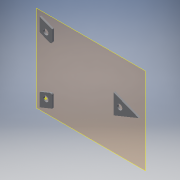
# Autodesk Inventor part: Orelhinhas
Saved by Autodesk Inventor 2019 (Build 230136000, 136)
## iProperties
Created: 2020-05-31
Part Number: Orelhinhas
Material: Genérico
Document SubType Name: Modeling
Designer: lukas
Density: 1 g/cm^3
Appearance: Padrão
Categories: <MemberInstance><Categories><Category DisplayName="" Mnemonic="CABLEANDHARNESS" InternalName="e4a7e005-5e42-4d16-b293-125e7f0d0512"><Category DisplayName="" Mnemonic="CONNECTORS" InternalName="6f634eba-a678-4820-a31d-2c2d5ee6728e"><CategoryParameter DisplayName="" Mnemonic="REFDES" InternalName="c3740e8c-60ab-4d5d-8584-52b73222f2f0"/><Category DisplayName="" Mnemonic="DISCRETEWIRE" InternalName="9a3407de-09b2-4cdb-8c40-9708d5144a28"/></Category></Category></Categories><FamilyTemplate><FamilyTemplateParameters></FamilyTemplateParameters></FamilyTemplate><CategoryParameterMap><ParamToTemplateMap><ParamToTemplate CategoryParameter="//CategoryParameter[@InternalName='c3740e8c-60ab-4d5d-8584-52b73222f2f0']" ConstantValue=""/></ParamToTemplateMap></CategoryParameterMap></MemberInstance>
Author: lukas
Autodesk Inventor part; units mm, degrees
ref_plane "YZ Plane" through (0, 0, 0) normal (1, 0, 0) x (0, 1, 0)
ref_plane "XZ Plane" through (0, 0, 0) normal (0, 1, 0) x (-1, 0, 0)
ref_plane "XY Plane" through (0, 0, 0) normal (0, 0, 1) x (1, 0, 0)
ref_plane "Plano de trabalho1" through (0, 0, 0) normal (0, 0, 1) x (1, 0, 0)
sketch "Esboço1" plane through (0, 0, 0) normal (0, 0, 1) x (1, 0, 0)
  line L0 (69.9393, 0.6939) -> (-40.2626, 43.3703) projected
  line L1 (-40.2626, -44.0107) -> (69.9393, 0.6939) projected
  line L2 (-40.2626, 43.3703) -> (-40.2626, -44.0107) projected
  line L3 (-40.2626, 43.3703) -> (-26.2749, 37.9534)
  line L4 (-26.2749, 37.9534) -> (-26.2749, 25.8727)
  line L5 (-28.9971, 24.0077) -> (-38.9849, 27.8755)
  line L6 (-40.2626, 43.3703) -> (-40.2626, 29.7405)
  line L7 (-40.2626, -44.0107) -> (-26.3628, -38.372)
  line L8 (-26.3628, -38.372) -> (-26.3628, -26.3417)
  line L9 (-29.1146, -24.4883) -> (-39.0145, -28.5043)
  line L10 (-40.2626, -30.3576) -> (-40.2626, -44.0107)
  line L11 (69.9393, 0.6939) -> (41.9638, 11.5276)
  line L12 (41.9638, 11.5276) -> (41.9638, -10.6547)
  line L13 (69.9393, 0.6939) -> (41.9638, -10.6547)
  arc A0 (-28.9971, 24.0077) -> (-26.2749, 25.8727) centre (-28.2749, 25.8727) ccw
  arc A1 (-40.2626, 29.7405) -> (-38.9849, 27.8755) centre (-38.2626, 29.7405) ccw
  arc A2 (-26.3628, -26.3417) -> (-29.1146, -24.4883) centre (-28.3628, -26.3417) ccw
  arc A3 (-39.0145, -28.5043) -> (-40.2626, -30.3576) centre (-38.2626, -30.3576) ccw
  circle A4 centre (-33.3127, 31.9131) radius 3
  circle A5 centre (-33.3127, -32.3568) radius 3
  circle A6 centre (48.7636, 0.6939) radius 3
  point P0 (0, 0)
  point P1 (-26.2749, 22.9534)
  point P2 (-40.2626, 28.3703)
  point P3 (-26.3628, -23.372)
  point P4 (-40.2626, -29.0107)
  dimension "d0" = 15
  dimension "d1" = 15
  dimension "d2" = 15
  dimension "d3" = 15
  dimension "d4" = 15
  dimension "d5" = 30
  dimension "d6" = 2
  dimension "d7" = 6
  dimension "d8" = 6
  dimension "d9" = 6
  constraints: 22 end point, 14 point on line, 8 point on circle, 8 tangent, 7 centre point, 3 collinear, 3 equal radius, 2 parallel, 2 vertical
  measures "d0" distance of L0.end L3.end
  measures "d1" distance of L3.end point (-26.275, 22.953)
  measures "d2" distance of L1.start L7.end
  measures "d3" distance of L7.end point (-26.363, -23.372)
  measures "d4" distance of point (-26.363, -23.372) point (-40.263, -29.011)
  measures "d5" distance of L0.start L11.end
  measures "d6" radius of A0
  measures "d7" diameter of A4
  measures "d8" diameter of A5
  measures "d9" diameter of A6
extrude "Extrusão1" add sketch "Esboço1" along normal blind 2 contours L1 L12 L0 | L4 A0 L5 A1 L2 L0 | L1 L2 A3 L9 A2 L8
sketch "Esboço2" plane through (0, 0, 2) normal (0, 0, 1) x (1, 0, 0)
  circle A0 centre (-33.3127, -32.3568) radius 3 projected
